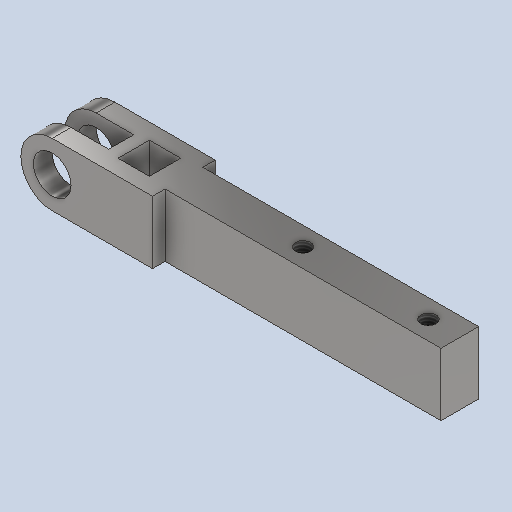
# Autodesk Inventor part: ramie
Saved by Autodesk Inventor 2022.1 (Build 261234020, 234B)
## iProperties
Created: 2022-05-02
Part Number: ramie
Material: Stal nierdzewna 440C
Document SubType Name: Modeling
Designer: Kacper Kaczmarski
Density: 7.75 g/cm^3
Appearance: Częściowo polerowany
Mass: 28.8377 g
Surface Area: 27.9683 cm^2
Volume: 3.72099 cm^3
Author: Kacper Kaczmarski
Autodesk Inventor part; units mm, degrees
ref_plane "YZ Plane" through (0, 0, 0) normal (1, 0, 0) x (0, 1, 0)
ref_plane "XZ Plane" through (0, 0, 0) normal (0, 1, 0) x (-1, 0, 0)
ref_plane "XY Plane" through (0, 0, 0) normal (0, 0, 1) x (1, 0, 0)
sketch "Szkic1" plane through (0, 0, 0) normal (0, 0, 1) x (1, 0, 0)
  line L0 (-16.906, 7.7541) -> (43.094, 7.7541)
  line L1 (43.094, 7.7541) -> (43.094, -2.2459)
  line L2 (43.094, -2.2459) -> (-16.906, -2.2459)
  line L3 (-16.906, -2.2459) -> (-16.906, 7.7541)
  arc A0 (-16.906, 7.7541) -> (-16.906, -2.2459) centre (-16.906, 2.7541) ccw
  circle A1 centre (-16.906, 2.7541) radius 3
  point P0 (0, 0)
  dimension "d0" = 60
  dimension "d1" = 10
  dimension "d2" = 6
  constraints: 8 end point, 2 centre point, 2 parallel, 2 point on circle, 2 tangent, 1 coincident, 1 horizontal, 1 perpendicular
  measures "d0" distance of L1.end L2.end
  measures "d1" distance of L0.end L1.end
  measures "d2" diameter of A1
extrude "Wyciągnięcie proste1" add sketch "Szkic1" along normal blind 10 contours L0 L1 L2 L3 A1 | L3 A1 A0
sketch "Szkic2" plane through (-16.906, -2.2459, 0) normal (0, -1, 0) x (1, 0, 0)
  line L0 (0, 0) -> (0, 10) projected
  line L1 (0, 5) -> (-8.6821, 5)
  line L2 (-8.6821, 5) -> (9.8833, 5)
  line L3 (-5, 0) -> (-5, 10) projected
  line L4 (-5, 7) -> (6, 7)
  line L5 (6, 7) -> (6, 3)
  line L6 (6, 3) -> (-5, 3)
  line L7 (-5, 3) -> (-5, 7)
  point P0 (16.906, 0)
  dimension "d5" = 11
  dimension "d6" = 4
  constraints: 12 end point, 2 horizontal, 2 parallel, 2 point on line, 1 midpoint, 1 perpendicular, 1 other
  measures "d5" distance of L5.end L6.end
  measures "d6" distance of L4.end L5.end
extrude "Wyciągnięcie proste2" cut sketch "Szkic2" against normal blind 10
sketch "Szkic3" plane through (-16.906, -2.2459, 0) normal (0, -1, 0) x (1, 0, 0)
  line L0 (0, 10) -> (60, 10) projected
  line L1 (8, 10) -> (8, 0)
  line L2 (6, 7) -> (6, 3) projected
  line L3 (13, 7.5) -> (8, 7.5)
  line L4 (8, 7.5) -> (8, 2.5)
  line L5 (8, 2.5) -> (13, 2.5)
  line L6 (13, 2.5) -> (13, 7.5)
  line L7 (6, 5) -> (16.5434, 5)
  point P0 (16.906, 0)
  dimension "d9" = 2
  dimension "d10" = 5
  dimension "d11" = 5
  constraints: 12 end point, 2 horizontal, 2 parallel, 2 perpendicular, 1 collinear, 1 midpoint, 1 point on line, 1 other
  measures "d9" distance between parallel lines of L1 L2
  measures "d10" distance of L5.end L4.end
  measures "d11" distance of L4.end L3.end
extrude "Wyciągnięcie proste3" cut sketch "Szkic3" against normal blind 10
sketch "Szkic4" plane through (-16.906, -2.2459, 0) normal (0, -1, 0) x (1, 0, 0)
  line L0 (60, 0) -> (60, 10) projected
  line L1 (60, 10) -> (16, 10)
  line L2 (16, 10) -> (16, 8)
  line L3 (16, 8) -> (60, 8)
  line L4 (60, 8) -> (60, 10)
  line L5 (60, 0) -> (0, 0) projected
  line L6 (60, 0) -> (16, 0)
  line L7 (16, 0) -> (16, 2)
  line L8 (16, 2) -> (60, 2)
  line L9 (60, 2) -> (60, 0)
  point P0 (16.906, 0)
  point P1 (16, 0)
  dimension "d14" = 44
  dimension "d15" = 2
  dimension "d16" = 44
  dimension "d17" = 2
  constraints: 16 end point, 4 parallel, 2 horizontal, 2 perpendicular
  measures "d14" distance of L3.end L2.end
  measures "d15" distance of L2.end L1.end
  measures "d16" distance of L7.end L8.end
  measures "d17" distance of L6.end L7.end
extrude "Wyciągnięcie proste4" cut sketch "Szkic4" against normal blind 10
sketch "Szkic5" plane through (-16.906, -2.2459, 7) normal (0, -1, 0) x (1, 0, 0)
  line L0 (16, 1) -> (60, 1) projected
  line L1 (30, 1) -> (30, -5.0068)
  line L2 (60, -5) -> (60, 1) projected
  line L3 (55, 1) -> (55, -5)
  line L4 (35, 1) -> (35, -5)
  line L5 (60, -5) -> (16, -5) projected
  line L6 (60, -2) -> (30, -2.0034)
  point P0 (16.906, -7)
  point P1 (55, -2.0006)
  point P2 (35, -2.0028)
  dimension "d20" = 30
  dimension "d21" = 5
  dimension "d22" = 25
  constraints: 8 end point, 8 point on line, 3 vertical, 2 midpoint
  measures "d20" distance between parallel lines of L1 L2
  measures "d21" distance between parallel lines of L3 L2
  measures "d22" distance between parallel lines of L4 L2
hole "Otwór1" at (38.094, -2.2459, 4.9994) at (18.094, -2.2459, 4.9972) direction (0, 1, 0) diameter 2.459 end through all thread size "M3x0.5" class "6H" standard "ISO Metric profile"
